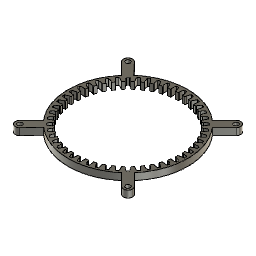
second_internal_gear_49.438mm_diameter v3 (Autodesk Fusion 360 design; units mm, degrees)
Autodesk Fusion 360 part; units mm, degrees
sketch "Sketch1" plane through (0, 0, 0) normal (0, 0, 1) x (1, 0, 0)
  spline S0 degree 5 poles (23.2193, -0.889) (23.2194, -0.889) (23.2195, -0.889) (23.2198, -0.889) (23.2203, -0.8891) (23.2209, -0.8891) (23.2217, -0.8891) (23.2226, -0.8891) (23.2235, -0.8891) (23.2246, -0.8891) (23.2257, -0.8892) (23.227, -0.8892) (23.2283, -0.8892) (23.2298, -0.8892) (23.2313, -0.8892) (23.2329, -0.8892) (23.2346, -0.8892) (23.2364, -0.8892) (23.2383, -0.8892) (23.2403, -0.8892) (23.2423, -0.8892) (23.2445, -0.8892) (23.2467, -0.8892) (23.249, -0.8891) (23.2514, -0.8891) (23.2539, -0.8891) (23.2565, -0.889) (23.2591, -0.889) (23.2618, -0.8889) (23.2646, -0.8888) (23.2675, -0.8888) (23.2704, -0.8887) (23.2735, -0.8886) (23.2766, -0.8885) (23.2798, -0.8884) (23.283, -0.8883) (23.2863, -0.8881) (23.2897, -0.888) (23.2932, -0.8879) (23.2968, -0.8877) (23.3004, -0.8876) (23.3041, -0.8874) (23.3079, -0.8872) (23.3117, -0.887) (23.3156, -0.8868) (23.3196, -0.8866) (23.3236, -0.8864) (23.3277, -0.8861) (23.3319, -0.8859) (23.3361, -0.8856) (23.3404, -0.8853) (23.3448, -0.8851) (23.3492, -0.8848) (23.3537, -0.8844) (23.3583, -0.8841) (23.3629, -0.8838) (23.3676, -0.8834) (23.3723, -0.8831) (23.3771, -0.8827) (23.382, -0.8823) (23.387, -0.8819) (23.3919, -0.8815) (23.397, -0.8811) (23.4021, -0.8806) (23.4073, -0.8802) (23.4125, -0.8797) (23.4178, -0.8792) (23.4232, -0.8787) (23.4286, -0.8782) (23.434, -0.8777) (23.4395, -0.8771) (23.4451, -0.8765) (23.4508, -0.876) (23.4564, -0.8754) (23.4622, -0.8748) (23.468, -0.8741) (23.4738, -0.8735) (23.4797, -0.8728) (23.4857, -0.8722) (23.4917, -0.8715) (23.4978, -0.8708) (23.5039, -0.87) (23.5101, -0.8693) (23.5163, -0.8685) (23.5225, -0.8678) (23.5289, -0.867) (23.5352, -0.8662) (23.5417, -0.8653) (23.5481, -0.8645) (23.5547, -0.8636) (23.5612, -0.8628) (23.5679, -0.8619) (23.5745, -0.8609) (23.5813, -0.86) (23.588, -0.8591) (23.5948, -0.8581) (23.6017, -0.8571) (23.6086, -0.8561) (23.6156, -0.8551) (23.6226, -0.854) (23.6296, -0.853) (23.6367, -0.8519) (23.6439, -0.8508) (23.6511, -0.8497) (23.6583, -0.8485) (23.6656, -0.8474) (23.6729, -0.8462) (23.6803, -0.845) (23.6877, -0.8438) (23.6951, -0.8425) (23.7026, -0.8413) (23.7102, -0.84) (23.7178, -0.8387) (23.7254, -0.8374) (23.7331, -0.8361) (23.7408, -0.8347) (23.7485, -0.8334) (23.7563, -0.832) (23.7642, -0.8305) (23.7721, -0.8291) (23.78, -0.8277) (23.788, -0.8262) (23.796, -0.8247) (23.804, -0.8232) (23.8121, -0.8216) (23.8202, -0.8201) (23.8284, -0.8185) (23.8366, -0.8169) (23.8448, -0.8153) (23.8531, -0.8136) (23.8614, -0.812) (23.8698, -0.8103) (23.8782, -0.8086) (23.8866, -0.8069) (23.8951, -0.8051) (23.9036, -0.8033) (23.9122, -0.8015) (23.9208, -0.7997) (23.9294, -0.7979) (23.9381, -0.796) (23.9468, -0.7942) (23.9555, -0.7923) (23.9643, -0.7903) (23.9731, -0.7884) (23.9819, -0.7864) (23.9908, -0.7844) (23.9997, -0.7824) (24.0087, -0.7804) (24.0176, -0.7783) (24.0267, -0.7763) (24.0357, -0.7742) (24.0448, -0.7721) (24.0539, -0.7699) (24.0631, -0.7677) (24.0723, -0.7656) (24.0815, -0.7633) (24.0908, -0.7611) (24.1001, -0.7588) (24.1094, -0.7566) (24.1188, -0.7543) (24.1282, -0.7519) (24.1376, -0.7496) (24.147, -0.7472) (24.1565, -0.7448) (24.1661, -0.7424) (24.1756, -0.74) (24.1852, -0.7375) (24.1948, -0.735) (24.2045, -0.7325) (24.2141, -0.73) (24.2239, -0.7274) (24.2336, -0.7248) (24.2434, -0.7222) (24.2532, -0.7196) (24.263, -0.717) (24.2729, -0.7143) (24.2828, -0.7116) (24.2927, -0.7089) (24.3027, -0.7061) (24.3126, -0.7033) (24.3227, -0.7006) (24.3327, -0.6977) (24.3428, -0.6949) (24.3529, -0.692) (24.363, -0.6891) (24.3732, -0.6862) (24.3834, -0.6833) (24.3936, -0.6803) (24.4038, -0.6774) (24.4141, -0.6743) (24.4244, -0.6713) (24.4347, -0.6683) (24.4451, -0.6652) (24.4555, -0.6621) (24.4659, -0.6589) (24.4763, -0.6558) (24.4868, -0.6526) (24.4973, -0.6494) (24.5078, -0.6462) (24.5184, -0.6429) (24.529, -0.6396) (24.5396, -0.6363) (24.5502, -0.633) (24.5608, -0.6297) (24.5715, -0.6263) (24.5822, -0.6229) (24.593, -0.6195) (24.6037, -0.616) (24.6145, -0.6126) (24.6253, -0.6091) (24.6361, -0.6055) (24.647, -0.602) (24.6579, -0.5984) (24.6688, -0.5948) (24.6797, -0.5912) (24.6907, -0.5875) (24.7017, -0.5839) (24.7127, -0.5802) (24.7237, -0.5764) (24.7348, -0.5727) (24.7458, -0.5689) (24.7569, -0.5651) (24.7681, -0.5613) (24.7792, -0.5575) (24.7904, -0.5536) (24.8016, -0.5497) (24.8128, -0.5458) (24.8241, -0.5418) (24.8353, -0.5378) (24.8466, -0.5338) (24.8579, -0.5298) (24.8693, -0.5258) (24.8806, -0.5217) (24.892, -0.5176) (24.9034, -0.5135) (24.9148, -0.5093) (24.9263, -0.5051) (24.9377, -0.5009) (24.9492, -0.4967) (24.9607, -0.4924) (24.9723, -0.4882) (24.9815, -0.4847) (24.9885, -0.4821) (24.9931, -0.4804) (24.9954, -0.4795) knots 0 0 0 0 0 0 0.00416667 0.00833333 0.0125 0.01666667 0.02083333 0.025 0.02916667 0.03333333 0.0375 0.04166667 0.04583333 0.05 0.05416667 0.05833333 0.0625 0.06666667 0.07083333 0.075 0.07916667 0.08333333 0.0875 0.09166667 0.09583333 0.1 0.10416667 0.10833333 0.1125 0.11666667 0.12083333 0.125 0.12916667 0.13333333 0.1375 0.14166667 0.14583333 0.15 0.15416667 0.15833333 0.1625 0.16666667 0.17083333 0.175 0.17916667 0.18333333 0.1875 0.19166667 0.19583333 0.2 0.20416667 0.20833333 0.2125 0.21666667 0.22083333 0.225 0.22916667 0.23333333 0.2375 0.24166667 0.24583333 0.25 0.25416667 0.25833333 0.2625 0.26666667 0.27083333 0.275 0.27916667 0.28333333 0.2875 0.29166667 0.29583333 0.3 0.30416667 0.30833333 0.3125 0.31666667 0.32083333 0.325 0.32916667 0.33333333 0.3375 0.34166667 0.34583333 0.35 0.35416667 0.35833333 0.3625 0.36666667 0.37083333 0.375 0.37916667 0.38333333 0.3875 0.39166667 0.39583333 0.4 0.40416667 0.40833333 0.4125 0.41666667 0.42083333 0.425 0.42916667 0.43333333 0.4375 0.44166667 0.44583333 0.45 0.45416667 0.45833333 0.4625 0.46666667 0.47083333 0.475 0.47916667 0.48333333 0.4875 0.49166667 0.49583333 0.5 0.50416667 0.50833333 0.5125 0.51666667 0.52083333 0.525 0.52916667 0.53333333 0.5375 0.54166667 0.54583333 0.55 0.55416667 0.55833333 0.5625 0.56666667 0.57083333 0.575 0.57916667 0.58333333 0.5875 0.59166667 0.59583333 0.6 0.60416667 0.60833333 0.6125 0.61666667 0.62083333 0.625 0.62916667 0.63333333 0.6375 0.64166667 0.64583333 0.65 0.65416667 0.65833333 0.6625 0.66666667 0.67083333 0.675 0.67916667 0.68333333 0.6875 0.69166667 0.69583333 0.7 0.70416667 0.70833333 0.7125 0.71666667 0.72083333 0.725 0.72916667 0.73333333 0.7375 0.74166667 0.74583333 0.75 0.75416667 0.75833333 0.7625 0.76666667 0.77083333 0.775 0.77916667 0.78333333 0.7875 0.79166667 0.79583333 0.8 0.80416667 0.80833333 0.8125 0.81666667 0.82083333 0.825 0.82916667 0.83333333 0.8375 0.84166667 0.84583333 0.85 0.85416667 0.85833333 0.8625 0.86666667 0.87083333 0.875 0.87916667 0.88333333 0.8875 0.89166667 0.89583333 0.9 0.90416667 0.90833333 0.9125 0.91666667 0.92083333 0.925 0.92916667 0.93333333 0.9375 0.94166667 0.94583333 0.95 0.95416667 0.95833333 0.9625 0.96666667 0.97083333 0.975 0.97916667 0.98333333 0.9875 0.99166667 0.99583333 1 1 1 1 1 1
  spline S1 degree 5 poles (23.2193, 0.889) (23.2194, 0.889) (23.2195, 0.889) (23.2198, 0.889) (23.2203, 0.8891) (23.2209, 0.8891) (23.2217, 0.8891) (23.2226, 0.8891) (23.2235, 0.8891) (23.2246, 0.8891) (23.2257, 0.8892) (23.227, 0.8892) (23.2283, 0.8892) (23.2298, 0.8892) (23.2313, 0.8892) (23.2329, 0.8892) (23.2346, 0.8892) (23.2364, 0.8892) (23.2383, 0.8892) (23.2403, 0.8892) (23.2423, 0.8892) (23.2445, 0.8892) (23.2467, 0.8892) (23.249, 0.8891) (23.2514, 0.8891) (23.2539, 0.8891) (23.2565, 0.889) (23.2591, 0.889) (23.2618, 0.8889) (23.2646, 0.8888) (23.2675, 0.8888) (23.2704, 0.8887) (23.2735, 0.8886) (23.2766, 0.8885) (23.2798, 0.8884) (23.283, 0.8883) (23.2863, 0.8881) (23.2897, 0.888) (23.2932, 0.8879) (23.2968, 0.8877) (23.3004, 0.8876) (23.3041, 0.8874) (23.3079, 0.8872) (23.3117, 0.887) (23.3156, 0.8868) (23.3196, 0.8866) (23.3236, 0.8864) (23.3277, 0.8861) (23.3319, 0.8859) (23.3361, 0.8856) (23.3404, 0.8853) (23.3448, 0.8851) (23.3492, 0.8848) (23.3537, 0.8844) (23.3583, 0.8841) (23.3629, 0.8838) (23.3676, 0.8834) (23.3723, 0.8831) (23.3771, 0.8827) (23.382, 0.8823) (23.387, 0.8819) (23.3919, 0.8815) (23.397, 0.8811) (23.4021, 0.8806) (23.4073, 0.8802) (23.4125, 0.8797) (23.4178, 0.8792) (23.4232, 0.8787) (23.4286, 0.8782) (23.434, 0.8777) (23.4395, 0.8771) (23.4451, 0.8765) (23.4508, 0.876) (23.4564, 0.8754) (23.4622, 0.8748) (23.468, 0.8741) (23.4738, 0.8735) (23.4797, 0.8728) (23.4857, 0.8722) (23.4917, 0.8715) (23.4978, 0.8708) (23.5039, 0.87) (23.5101, 0.8693) (23.5163, 0.8685) (23.5225, 0.8678) (23.5289, 0.867) (23.5352, 0.8662) (23.5417, 0.8653) (23.5481, 0.8645) (23.5547, 0.8636) (23.5612, 0.8628) (23.5679, 0.8619) (23.5745, 0.8609) (23.5813, 0.86) (23.588, 0.8591) (23.5948, 0.8581) (23.6017, 0.8571) (23.6086, 0.8561) (23.6156, 0.8551) (23.6226, 0.854) (23.6296, 0.853) (23.6367, 0.8519) (23.6439, 0.8508) (23.6511, 0.8497) (23.6583, 0.8485) (23.6656, 0.8474) (23.6729, 0.8462) (23.6803, 0.845) (23.6877, 0.8438) (23.6951, 0.8425) (23.7026, 0.8413) (23.7102, 0.84) (23.7178, 0.8387) (23.7254, 0.8374) (23.7331, 0.8361) (23.7408, 0.8347) (23.7485, 0.8334) (23.7563, 0.832) (23.7642, 0.8305) (23.7721, 0.8291) (23.78, 0.8277) (23.788, 0.8262) (23.796, 0.8247) (23.804, 0.8232) (23.8121, 0.8216) (23.8202, 0.8201) (23.8284, 0.8185) (23.8366, 0.8169) (23.8448, 0.8153) (23.8531, 0.8136) (23.8614, 0.812) (23.8698, 0.8103) (23.8782, 0.8086) (23.8866, 0.8069) (23.8951, 0.8051) (23.9036, 0.8033) (23.9122, 0.8015) (23.9208, 0.7997) (23.9294, 0.7979) (23.9381, 0.796) (23.9468, 0.7942) (23.9555, 0.7923) (23.9643, 0.7903) (23.9731, 0.7884) (23.9819, 0.7864) (23.9908, 0.7844) (23.9997, 0.7824) (24.0087, 0.7804) (24.0176, 0.7783) (24.0267, 0.7763) (24.0357, 0.7742) (24.0448, 0.7721) (24.0539, 0.7699) (24.0631, 0.7677) (24.0723, 0.7656) (24.0815, 0.7633) (24.0908, 0.7611) (24.1001, 0.7588) (24.1094, 0.7566) (24.1188, 0.7543) (24.1282, 0.7519) (24.1376, 0.7496) (24.147, 0.7472) (24.1565, 0.7448) (24.1661, 0.7424) (24.1756, 0.74) (24.1852, 0.7375) (24.1948, 0.735) (24.2045, 0.7325) (24.2141, 0.73) (24.2239, 0.7274) (24.2336, 0.7248) (24.2434, 0.7222) (24.2532, 0.7196) (24.263, 0.717) (24.2729, 0.7143) (24.2828, 0.7116) (24.2927, 0.7089) (24.3027, 0.7061) (24.3126, 0.7033) (24.3227, 0.7006) (24.3327, 0.6977) (24.3428, 0.6949) (24.3529, 0.692) (24.363, 0.6891) (24.3732, 0.6862) (24.3834, 0.6833) (24.3936, 0.6803) (24.4038, 0.6774) (24.4141, 0.6743) (24.4244, 0.6713) (24.4347, 0.6683) (24.4451, 0.6652) (24.4555, 0.6621) (24.4659, 0.6589) (24.4763, 0.6558) (24.4868, 0.6526) (24.4973, 0.6494) (24.5078, 0.6462) (24.5184, 0.6429) (24.529, 0.6396) (24.5396, 0.6363) (24.5502, 0.633) (24.5608, 0.6297) (24.5715, 0.6263) (24.5822, 0.6229) (24.593, 0.6195) (24.6037, 0.616) (24.6145, 0.6126) (24.6253, 0.6091) (24.6361, 0.6055) (24.647, 0.602) (24.6579, 0.5984) (24.6688, 0.5948) (24.6797, 0.5912) (24.6907, 0.5875) (24.7017, 0.5839) (24.7127, 0.5802) (24.7237, 0.5764) (24.7348, 0.5727) (24.7458, 0.5689) (24.7569, 0.5651) (24.7681, 0.5613) (24.7792, 0.5575) (24.7904, 0.5536) (24.8016, 0.5497) (24.8128, 0.5458) (24.8241, 0.5418) (24.8353, 0.5378) (24.8466, 0.5338) (24.8579, 0.5298) (24.8693, 0.5258) (24.8806, 0.5217) (24.892, 0.5176) (24.9034, 0.5135) (24.9148, 0.5093) (24.9263, 0.5051) (24.9377, 0.5009) (24.9492, 0.4967) (24.9607, 0.4924) (24.9723, 0.4882) (24.9815, 0.4847) (24.9885, 0.4821) (24.9931, 0.4804) (24.9954, 0.4795) knots 0 0 0 0 0 0 0.00416667 0.00833333 0.0125 0.01666667 0.02083333 0.025 0.02916667 0.03333333 0.0375 0.04166667 0.04583333 0.05 0.05416667 0.05833333 0.0625 0.06666667 0.07083333 0.075 0.07916667 0.08333333 0.0875 0.09166667 0.09583333 0.1 0.10416667 0.10833333 0.1125 0.11666667 0.12083333 0.125 0.12916667 0.13333333 0.1375 0.14166667 0.14583333 0.15 0.15416667 0.15833333 0.1625 0.16666667 0.17083333 0.175 0.17916667 0.18333333 0.1875 0.19166667 0.19583333 0.2 0.20416667 0.20833333 0.2125 0.21666667 0.22083333 0.225 0.22916667 0.23333333 0.2375 0.24166667 0.24583333 0.25 0.25416667 0.25833333 0.2625 0.26666667 0.27083333 0.275 0.27916667 0.28333333 0.2875 0.29166667 0.29583333 0.3 0.30416667 0.30833333 0.3125 0.31666667 0.32083333 0.325 0.32916667 0.33333333 0.3375 0.34166667 0.34583333 0.35 0.35416667 0.35833333 0.3625 0.36666667 0.37083333 0.375 0.37916667 0.38333333 0.3875 0.39166667 0.39583333 0.4 0.40416667 0.40833333 0.4125 0.41666667 0.42083333 0.425 0.42916667 0.43333333 0.4375 0.44166667 0.44583333 0.45 0.45416667 0.45833333 0.4625 0.46666667 0.47083333 0.475 0.47916667 0.48333333 0.4875 0.49166667 0.49583333 0.5 0.50416667 0.50833333 0.5125 0.51666667 0.52083333 0.525 0.52916667 0.53333333 0.5375 0.54166667 0.54583333 0.55 0.55416667 0.55833333 0.5625 0.56666667 0.57083333 0.575 0.57916667 0.58333333 0.5875 0.59166667 0.59583333 0.6 0.60416667 0.60833333 0.6125 0.61666667 0.62083333 0.625 0.62916667 0.63333333 0.6375 0.64166667 0.64583333 0.65 0.65416667 0.65833333 0.6625 0.66666667 0.67083333 0.675 0.67916667 0.68333333 0.6875 0.69166667 0.69583333 0.7 0.70416667 0.70833333 0.7125 0.71666667 0.72083333 0.725 0.72916667 0.73333333 0.7375 0.74166667 0.74583333 0.75 0.75416667 0.75833333 0.7625 0.76666667 0.77083333 0.775 0.77916667 0.78333333 0.7875 0.79166667 0.79583333 0.8 0.80416667 0.80833333 0.8125 0.81666667 0.82083333 0.825 0.82916667 0.83333333 0.8375 0.84166667 0.84583333 0.85 0.85416667 0.85833333 0.8625 0.86666667 0.87083333 0.875 0.87916667 0.88333333 0.8875 0.89166667 0.89583333 0.9 0.90416667 0.90833333 0.9125 0.91666667 0.92083333 0.925 0.92916667 0.93333333 0.9375 0.94166667 0.94583333 0.95 0.95416667 0.95833333 0.9625 0.96666667 0.97083333 0.975 0.97916667 0.98333333 0.9875 0.99166667 0.99583333 1 1 1 1 1 1
  spline S2 degree 5 poles (23.2185, -0.889) (23.2186, -0.889) (23.2186, -0.889) (23.2187, -0.889) (23.2188, -0.889) (23.219, -0.889) (23.2191, -0.889) (23.2192, -0.889) (23.2193, -0.889) (23.2193, -0.889) knots 0 0 0 0 0 0 0.2 0.4 0.6 0.8 1 1 1 1 1 1
  spline S3 degree 5 poles (23.2185, 0.889) (23.2186, 0.889) (23.2186, 0.889) (23.2187, 0.889) (23.2188, 0.889) (23.219, 0.889) (23.2191, 0.889) (23.2192, 0.889) (23.2193, 0.889) (23.2193, 0.889) knots 0 0 0 0 0 0 0.2 0.4 0.6 0.8 1 1 1 1 1 1
  line L0 (0, 0) -> (23.2185, -0.889)
  line L1 (0, 0) -> (23.2185, 0.889)
  arc A0 (24.9954, -0.4795) -> (24.9954, 0.4795) centre (0, 0) ccw
  point P0 (23.2216, -0.8891)
  point P1 (23.2254, -0.8892)
  point P2 (23.2307, -0.8892)
  point P3 (23.2376, -0.8892)
  point P4 (23.246, -0.8892)
  point P5 (23.2559, -0.889)
  point P6 (23.2673, -0.8888)
  point P7 (23.2803, -0.8884)
  point P8 (23.2948, -0.8878)
  point P9 (23.3108, -0.8871)
  point P10 (23.3283, -0.8861)
  point P11 (23.3473, -0.8849)
  point P12 (23.3679, -0.8834)
  point P13 (23.3899, -0.8817)
  point P14 (23.4135, -0.8796)
  point P15 (23.4385, -0.8772)
  point P16 (23.4651, -0.8744)
  point P17 (23.4931, -0.8713)
  point P18 (23.5227, -0.8677)
  point P19 (23.5537, -0.8638)
  point P20 (23.5862, -0.8593)
  point P21 (23.6202, -0.8544)
  point P22 (23.6556, -0.8489)
  point P23 (23.6925, -0.843)
  point P24 (23.7309, -0.8365)
  point P25 (23.7707, -0.8294)
  point P26 (23.8119, -0.8217)
  point P27 (23.8546, -0.8133)
  point P28 (23.8987, -0.8044)
  point P29 (23.9442, -0.7947)
  point P30 (23.9911, -0.7844)
  point P31 (24.0394, -0.7733)
  point P32 (24.0892, -0.7615)
  point P33 (24.1403, -0.7489)
  point P34 (24.1928, -0.7355)
  point P35 (24.2466, -0.7214)
  point P36 (24.3018, -0.7063)
  point P37 (24.3584, -0.6905)
  point P38 (24.4162, -0.6737)
  point P39 (24.4754, -0.6561)
  point P40 (24.536, -0.6375)
  point P41 (24.5978, -0.6179)
  point P42 (24.6609, -0.5974)
  point P43 (24.7253, -0.5759)
  point P44 (24.791, -0.5534)
  point P45 (24.8579, -0.5298)
  point P46 (24.926, -0.5052)
  point P47 (23.2216, 0.8891)
  point P48 (23.2254, 0.8892)
  point P49 (23.2307, 0.8892)
  point P50 (23.2376, 0.8892)
  point P51 (23.246, 0.8892)
  point P52 (23.2559, 0.889)
  point P53 (23.2673, 0.8888)
  point P54 (23.2803, 0.8884)
  point P55 (23.2948, 0.8878)
  point P56 (23.3108, 0.8871)
  point P57 (23.3283, 0.8861)
  point P58 (23.3473, 0.8849)
  point P59 (23.3679, 0.8834)
  point P60 (23.3899, 0.8817)
  point P61 (23.4135, 0.8796)
  point P62 (23.4385, 0.8772)
  point P63 (23.4651, 0.8744)
  point P64 (23.4931, 0.8713)
  point P65 (23.5227, 0.8677)
  point P66 (23.5537, 0.8638)
  point P67 (23.5862, 0.8593)
  point P68 (23.6202, 0.8544)
  point P69 (23.6556, 0.8489)
  point P70 (23.6925, 0.843)
  point P71 (23.7309, 0.8365)
  point P72 (23.7707, 0.8294)
  point P73 (23.8119, 0.8217)
  point P74 (23.8546, 0.8133)
  point P75 (23.8987, 0.8044)
  point P76 (23.9442, 0.7947)
  point P77 (23.9911, 0.7844)
  point P78 (24.0394, 0.7733)
  point P79 (24.0892, 0.7615)
  point P80 (24.1403, 0.7489)
  point P81 (24.1928, 0.7355)
  point P82 (24.2466, 0.7214)
  point P83 (24.3018, 0.7063)
  point P84 (24.3584, 0.6905)
  point P85 (24.4162, 0.6737)
  point P86 (24.4754, 0.6561)
  point P87 (24.536, 0.6375)
  point P88 (24.5978, 0.6179)
  point P89 (24.6609, 0.5974)
  point P90 (24.7253, 0.5759)
  point P91 (24.791, 0.5534)
  point P92 (24.8579, 0.5298)
  point P93 (24.926, 0.5052)
sketch "Sketch2" plane through (0, 0, 0) normal (0, 0, 1) x (1, 0, 0)
  circle A0 centre (0, 0) radius 26
  circle A1 centre (0, 0) radius 22.75
  circle A2 centre (0, 0) radius 22.75
extrude "Extrude1" add sketch "Sketch2" along normal blind 3
extrude "Extrude2" cut sketch "Sketch1" along normal blind 3
pattern_circular "C-Pattern1" count 48 over 360 about axis through (0, 0, 1.75) along (0, 0, 1) of "Extrude2"
sketch "Sketch3" plane through (0, 0, 0) normal (0, 0, 1) x (1, 0, 0)
  line L0 (0, 0) -> (46.2012, 0) construction
  line L1 (46.2012, 0) -> (46.2012, 3) construction
  line L2 (46.2012, 3) -> (0, 3) construction
  line L3 (0, 3) -> (0, 0) construction
  constraint perpendicular L0 L1
  constraint parallel L0 L2
  constraint parallel L1 L3
sketch "Sketch4" plane through (0, 0, 0) normal (0, 0, 1) x (1, 0, 0)
  circle A0 centre (0, 0) radius 35.5
  line L0 (0, 0) -> (33.25, 0) construction
  circle A1 centre (-23.5113, 23.5113) radius 1
  circle A2 centre (23.5113, 23.5113) radius 1
  circle A3 centre (-23.5113, -23.5113) radius 1
  circle A4 centre (23.5113, -23.5113) radius 1
  line L1 (-18, -18) -> (-18.0708, -18)
  line L2 (-17.3283, -18.7425) -> (-19.124, -16.9468)
  line L3 (-17.3283, -18.7425) -> (-16.8587, -19.2121)
  line L4 (-22.0971, -24.9255) -> (-16.8587, -19.2121)
  line L5 (-24.9255, -22.0971) -> (-19.4369, -16.6085)
  line L6 (-19.4369, -16.6085) -> (-19.124, -16.9468)
  line L7 (-23.7876, -22.5502) -> (-24.2184, -22.8042)
  arc A5 (-24.9255, -22.0971) -> (-21.98, -24.7978) centre (-23.5113, -23.5113) ccw
  line L8 (0, 0) -> (-18.0354, -18.0354)
  line L9 (-22.8042, -22.8042) -> (-23.5113, -23.5113)
  line L10 (-18, -18.0708) -> (-18, -18)
  line L11 (-24.9255, 22.0971) -> (-19.2936, 16.4652)
  line L12 (-22.0971, 24.9255) -> (-16.5, 19)
  line L13 (-16.5, 19) -> (-19.2936, 16.4652)
  arc A6 (-22.0188, 24.8427) -> (-24.9255, 22.0971) centre (-23.5113, 23.5113) ccw
  line L14 (22.0971, 24.9255) -> (16.5975, 19.426)
  line L15 (24.9255, 22.0971) -> (19.4378, 16.6094)
  line L16 (19.4378, 16.6094) -> (16.5975, 19.426)
  arc A7 (24.9255, 22.0971) -> (22.0971, 24.9255) centre (23.5113, 23.5113) ccw
  line L17 (0, 0) -> (18.0177, 18.0177)
  line L18 (24.9255, -22.0971) -> (19.3686, -16.5402)
  line L19 (22.0971, -24.9255) -> (16.3818, -19.2103)
  line L20 (16.3818, -19.2103) -> (19.3686, -16.5402)
  arc A8 (22.0971, -24.9255) -> (24.9255, -22.0971) centre (23.5113, -23.5113) ccw
  line L21 (0, 0) -> (17.8752, -17.8752)
  dimension "d7" = 71
  dimension "d9" = 45
  dimension "d10" = 2
  dimension "d11" = 2
  dimension "d12" = 2
  dimension "d13" = 2
  dimension "d15" = 1
  constraint coincident A0.centre L0.start
  constraint horizontal L0
  constraint perpendicular L17 L21
  constraint perpendicular L8 L21
  constraint coincident A3.centre A5.centre
  constraint coincident A3 L7.end
  constraint horizontal L1
  constraint coincident L1.start L8
  constraint concentric A3 A5
  constraint coincident A3 L7.start
  constraint coincident L4 A5.end
  constraint coincident A3 L9.start
  constraint collinear L8 L9
  constraint coincident L2 L8.end
  constraint coincident L2 L1.end
  constraint coincident L2 L10.start
  constraint concentric A1 A6
  constraint coincident L12.start A6
  constraint tangent L11 A6
  constraint coincident L12 A6.start
  constraint concentric A2 A7
  constraint tangent L14 A7
  constraint tangent L15 A7
  constraint coincident L16 L17.end
  constraint concentric A4 A8
  constraint tangent L18 A8
  constraint tangent L19 A8
  constraint coincident L20 L21.end
  measures "d7" diameter of A0
  measures "d9" angle of L0 L17
  measures "d10" diameter of A1
  measures "d11" diameter of A2
  measures "d12" diameter of A3
  measures "d13" diameter of A4
  measures "d15" distance of L7.end L5.start
extrude "Extrude3" add sketch "Sketch4" along normal blind 3 contours L2 L3 L4 L5 L6 A5 | L11 L12 L13 A6 | L14 L15 L16 A7 | L18 L19 L20 A8
